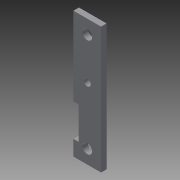
# Autodesk Inventor part: m
Saved by Autodesk Inventor 2015 (Build 190159000, 159)
## iProperties
Created: 2015-11-06
Part Number: m
Material: Generic
Document SubType Name: Modeling
Designer: EriveltonDell
Density: 1 g/cm^3
Appearance: Default
Author: EriveltonDell
Autodesk Inventor part; units mm, degrees
ref_plane "YZ Plane" through (0, 0, 0) normal (1, 0, 0) x (0, 1, 0)
ref_plane "XZ Plane" through (0, 0, 0) normal (0, 1, 0) x (-1, 0, 0)
ref_plane "XY Plane" through (0, 0, 0) normal (0, 0, 1) x (1, 0, 0)
sketch "Sketch1" plane through (0, 0, 0) normal (0, 1, 0) x (-1, 0, 0)
  circle A0 centre (0, 0) radius 10.5
  line L0 (0, 0) -> (0, -23.5)
  circle A1 centre (0, -23.5) radius 5.25
  line L1 (0, -23.5) -> (0, -35.25)
  line L2 (-14, -35.25) -> (-14, -58.75)
  line L3 (-14, -58.75) -> (-19, -58.75)
  line L4 (-19, -58.75) -> (-19, -35.25)
  line L5 (-35.25, 21.625) -> (35.25, 21.625) construction
  line L6 (35.25, 21.625) -> (25.25, 21.625)
  line L7 (-35.25, -69.875) -> (-35.25, 21.625)
  line L8 (-35.25, 21.625) -> (-35.25, 11.625)
  line L9 (-35.25, 11.625) -> (-25.25, 11.625)
  circle A2 centre (-25.25, 11.625) radius 3.5
  line L10 (35.25, 21.625) -> (25.25, 21.625)
  line L11 (25.25, 21.625) -> (25.25, 11.625)
  circle A3 centre (25.25, 11.625) radius 3.5
  line L12 (35.25, -69.875) -> (25.25, -69.875)
  line L13 (25.25, -69.875) -> (25.25, -59.875)
  circle A4 centre (25.25, -59.875) radius 3.5
  line L14 (-35.25, -69.875) -> (-25.25, -69.875)
  line L15 (-25.25, -69.875) -> (-25.25, -59.875)
  circle A5 centre (-25.25, -59.875) radius 3.5
  line L16 (-25.25, 11.625) -> (-25.25, -18.375)
  circle A6 centre (-25.25, -18.375) radius 2.5
  circle A7 centre (25.25, -29.875) radius 2.5
  line L17 (-19, -35.25) -> (-14, -35.25)
  line L18 (-35.25, 21.625) -> (-15.25, 21.625)
  line L19 (35.25, 21.625) -> (35.25, 11.625)
  line L20 (35.25, -58.75) -> (35.25, -69.875)
  line L21 (35.25, -69.875) -> (25.25, -69.875)
  line L22 (-15.25, -69.875) -> (-35.25, -69.875)
  line L23 (-35.25, 21.625) -> (-15.25, 21.625)
  line L24 (25.25, 21.625) -> (35.25, 21.625)
  line L25 (-35.25, 21.625) -> (-15.25, 21.625)
  line L26 (25.25, 21.625) -> (35.25, 21.625)
  line L27 (25.25, -59.875) -> (25.25, -56.375)
  line L28 (25.25, -32.375) -> (25.25, -29.875)
  line L29 (-15.25, 21.625) -> (-15.25, -35.25)
  line L30 (-15.25, -58.75) -> (-15.25, -69.875)
  dimension "d53" = 7
  dimension "d63" = 5
  dimension "d0" = 21
  dimension "d1" = 23.5
  dimension "d2" = 10.5
  dimension "d3" = 11.75
  dimension "d5" = 23.5
  dimension "d6" = 5
  dimension "d7" = 23.5
  dimension "d9" = 70.5
  dimension "d41" = 70.5
  dimension "d42" = 91.5
  dimension "d43" = 10
  dimension "d44" = 10
  dimension "d45" = 7
  dimension "d46" = 10
  dimension "d47" = 10
  dimension "d48" = 90
  dimension "d50" = 7
  dimension "d51" = 10
  dimension "d52" = 10
  dimension "d54" = 10
  dimension "d55" = 10
  dimension "d56" = 7
  dimension "d60" = 30
  dimension "d61" = 30
  dimension "d62" = 5
  dimension "d65" = 20
  constraints: 62 end point, 13 perpendicular, 8 coincident, 6 centre point, 6 horizontal, 6 parallel, 6 point on line, 5 vertical, 2 vertical alignment, 1 collinear, 1 midpoint, 4 other
  measures "d0" diameter of A0
  measures "d1" distance of L0.start L0.end
  measures "d2" diameter of A1
  measures "d3" distance of L1.start L1.end
  measures "d5" distance of L2.start L2.end
  measures "d6" distance of L2.end L3.end
  measures "d7" distance of L3.end L4.end
  measures "d9" distance of L5.start L26.end
  measures "d41" distance of L12.start L7.start
  measures "d42" distance of L10.start L12.start
  measures "d43" distance of L5.start L8.end
  measures "d44" distance of L8.end L9.end
  measures "d45" diameter of A2
  measures "d46" distance of L10.start L6.end
  measures "d47" distance of L6.end L11.end
  measures "d48" angle of L11 L10
  measures "d50" diameter of A3
  measures "d51" distance of L12.start L12.end
  measures "d52" distance of L12.end L13.end
  measures "d54" distance of L7.start L14.end
  measures "d55" distance of L14.end L15.end
  measures "d56" diameter of A5
  measures "d60" distance of L16.start L16.end
  measures "d61" distance of L27.start L28.end
  measures "d62" diameter of A6
  measures "d65" distance of L5.start L18.end
extrude "Extrusion1" add sketch "Sketch1" along normal blind 4 contours L17 L4 L3 L30 L22 L14 L7 L18 L29
body "Solid1"
